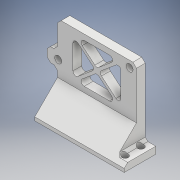
# Autodesk Inventor part: PingCover-y
Saved by Autodesk Inventor 2018.3 (Build 223284000, 284)
## iProperties
Created: 2018-08-25
Part Number: PingCover-y
Material: ABS プラスチック
Document SubType Name: Modeling
Designer: shun2
Density: 1.06 g/cm^3
Appearance: 滑らか - 白
Author: shun2
Autodesk Inventor part; units mm, degrees
sketch "スケッチ1" plane through (0, 0, 0) normal (0, 0, 1) x (1, 0, 0)
  line L0 (0, 0) -> (51, 0)
  line L1 (51, 0) -> (51, 18)
  line L2 (51, 18) -> (0, 18)
  line L3 (0, 18) -> (0, 0)
  circle A0 centre (47, 13.5) radius 1.8
  circle A1 centre (47, 4.5) radius 1.8
  dimension "d0" = 51
  dimension "d1" = 18
  dimension "d4" = 3.6
  dimension "d5" = 13.5
  dimension "d6" = 4
  dimension "d7" = 3.6
  dimension "d8" = 4
  dimension "d9" = 4.5
  constraints: 8 end point, 2 centre point, 2 parallel, 1 horizontal, 1 perpendicular
  measures "d0" distance of L2.end L1.end
  measures "d1" distance of L1.end L0.end
  measures "d4" diameter of A0
  measures "d5" distance from line of L0 A0.centre
  measures "d6" distance from line of L1 A0.centre
  measures "d7" diameter of A1
  measures "d8" distance from line of L1 A1.centre
  measures "d9" distance from line of L0 A1.centre
extrude "押し出し2" add sketch "スケッチ1" along normal blind 2
sketch "スケッチ2" plane through (0, 0, 2) normal (0, 0, 1) x (1, 0, 0)
  line L0 (0, 18) -> (0, 0) projected
  line L1 (0, 18) -> (44, 18)
  line L2 (44, 18) -> (44, 13)
  line L3 (44, 13) -> (0, 13)
  line L4 (0, 13) -> (0, 18)
  dimension "d12" = 44
  dimension "d13" = 5
  constraints: 8 end point, 2 parallel, 1 horizontal, 1 perpendicular
  measures "d12" distance of L2.end L3.end
  measures "d13" distance of L1.end L2.end
extrude "押し出し3" add sketch "スケッチ2" along normal blind 42
sketch "スケッチ3" plane through (0, 13, 2) normal (0, -1, 0) x (1, 0, 0)
  circle A0 centre (41.1, 3.5) radius 2
  line L0 (44, 0) -> (44, 42) projected
  line L1 (44, 0) -> (0, 0) projected
  circle A1 centre (0.4, 19.8) radius 2
  point P0 (0, -2)
  dimension "d16" = 4
  dimension "d17" = 2.9
  dimension "d18" = 3.5
  dimension "d27" = 4
  dimension "d28" = 40.7
  dimension "d29" = 16.3
  constraints: 2 centre point
  measures "d16" diameter of A0
  measures "d17" distance from line of L0 A0.centre
  measures "d18" distance from line of L1 A0.centre
  measures "d27" diameter of A1
  measures "d28" horizontal distance of A0.centre A1.centre
  measures "d29" vertical distance of A0.centre A1.centre
sketch "スケッチ4" plane through (0, 13, 2) normal (0, -1, 0) x (1, 0, 0)
  line L0 (8, 13.3) -> (-4, 13.3)
  line L1 (-4, 13.3) -> (-4, 24.3)
  line L2 (-4, 24.3) -> (8, 24.3)
  line L3 (8, 24.3) -> (8, 13.3)
  line L4 (44, 0) -> (0, 0) projected
  line L5 (44, 0) -> (44, 42) projected
  line L6 (0, 42) -> (44, 42) projected
  line L7 (0, 0) -> (0, 42) projected
  point P0 (0, -2)
  dimension "d19" = 13.3
  dimension "d20" = 36
  dimension "d25" = 11
  dimension "d26" = 12
  constraints: 8 end point, 2 parallel, 1 horizontal, 1 perpendicular
  measures "d19" distance between parallel lines of L0 L4
  measures "d20" distance between parallel lines of L5 L3
  measures "d25" distance between parallel lines of L0 L2
  measures "d26" distance between parallel lines of L1 L3
ref_plane "作業平面2" through (-4, 15.3, 26.3) normal (0, -1, 0) x (1, 0, 0)
sketch "スケッチ5" plane through (-4, 15.3, 26.3) normal (0, -1, 0) x (1, 0, 0)
  point P0 (4, -26.3)
ref_plane "作業平面1" through (-4, 15.3, 26.3) normal (0, -1, 0) x (1, 0, 0)
sketch "スケッチ6" plane through (-4, 15.3, 26.3) normal (0, -1, 0) x (1, 0, 0)
  line L0 (4, -24.3) -> (4, 17.7) projected
  circle A0 centre (4.4, -2.3) radius 2
  circle A1 centre (45.1, 14) radius 2
  line L1 (4, -24.3) -> (55, -24.3) projected
  line L2 (48, -24.3) -> (48, 17.7) projected
  line L3 (4, 17.7) -> (48, 17.7) projected
  point P0 (4, -26.3)
  dimension "d45" = 4
  dimension "d46" = 0.4
  dimension "d47" = 4
  dimension "d48" = 22
  dimension "d49" = 2.9
  dimension "d67" = 43.8427
  constraints: 2 centre point
  measures "d45" diameter of A0
  measures "d46" distance from line of L0 A0.centre
  measures "d47" diameter of A1
  measures "d48" distance from line of L1 A0.centre
  measures "d49" distance from line of L2 A1.centre
  measures "d67" distance of A0.centre A1.centre
sketch "スケッチ7" plane through (0, 13, 2) normal (0, -1, 0) x (1, 0, 0)
  point P0 (0, -2)
sketch "スケッチ8" plane through (0, 13, 2) normal (0, -1, 0) x (1, 0, 0)
  line L0 (44, 0) -> (44, 42) projected
  line L1 (44, 0) -> (45, 0)
  line L2 (45, 0) -> (45, 21.3)
  line L3 (45, 21.3) -> (44, 21.3)
  line L4 (44, 21.3) -> (44, 0)
  point P0 (0, -2)
  dimension "d35" = 1
  constraints: 8 end point, 2 parallel, 1 horizontal, 1 perpendicular
  measures "d35" distance of L3.end L2.end
extrude "押し出し6" add sketch "スケッチ8" against normal blind 5
ref_plane "作業平面3" through (45, 13, 3) normal (0, -1, 0) x (1, 0, 0)
sketch "スケッチ9" plane through (45, 13, 3) normal (0, -1, 0) x (1, 0, 0)
  line L0 (-51, 17.2309) -> (-43, 17.2309)
  line L1 (-43, 17.2309) -> (-43, 25.2309)
  line L2 (-43, 25.2309) -> (-51, 25.2309)
  line L3 (-51, 25.2309) -> (-51, 17.2309)
  line L4 (0, 41) -> (-10, 41)
  line L5 (-10, 41) -> (-10, 7.258)
  line L6 (-10, 7.258) -> (0, 7.258)
  line L7 (0, 7.258) -> (0, 41)
  line L8 (0, 16.7) -> (0, 41)
  line L9 (-45, -1) -> (6, -1) projected
  point P0 (-45, -3)
  point P1 (-45, 4.4596)
  point P2 (-2.5771, 20.3)
  dimension "d55" = 8
  dimension "d59" = 0
  dimension "d97" = 18.2309
  dimension "d98" = 8.258
  dimension "d99" = 33.742
  constraints: 18 end point, 2 parallel, 1 horizontal, 1 perpendicular
  measures "d55" distance between parallel lines of L0 L2
  measures "d59" distance between parallel lines of L8 L7
  measures "d97" distance between parallel lines of L0 L9
  measures "d98" distance between parallel lines of L6 L9
  measures "d99" distance between parallel lines of L4 L6
extrude "押し出し8" add sketch "スケッチ9" against normal blind 5
extrude "押し出し9" cut sketch "スケッチ6" along normal mid plane 10 contours A0 L0 | L0 A0 | A1
chamfer "面取り5" distance 13 angle 45 1 edges at (22.5, 13, 2)
sketch "スケッチ10" plane through (0, 0, 2) normal (0, 0, 1) x (1, 0, 0)
  line L0 (45, 18) -> (45, 0) projected
  line L1 (45, 0) -> (51, 0) projected
  line L2 (51, 0) -> (51, 18) projected
  line L3 (51, 18) -> (45, 18) projected
  circle A0 centre (47, 13.5) radius 1.8 projected
  circle A1 centre (47, 4.5) radius 1.8 projected
  circle A2 centre (47, 4.5) radius 1.8
  circle A3 centre (47, 13.5) radius 1.8
  line L4 (45, 0) -> (51, 0)
  line L5 (51, 0) -> (51, 18)
  line L6 (51, 18) -> (45, 18)
  line L7 (45, 18) -> (45, 0)
  point P0 (0, 0)
  constraints: 8 end point, 2 centre point, 2 coincident, 2 concentric, 2 parallel, 1 horizontal, 1 perpendicular
extrude "押し出し10" add sketch "スケッチ10" along normal blind 2
chamfer "面取り6" distance 2 angle 45 1 edges at (48, 0, 4)
chamfer "面取り7" distance 1.5 angle 45 1 edges at (45, 10.0001, 4)
chamfer "面取り8" distance 2 angle 45 4 edges at (45, 15.5, 44) (0, 15.5, 44) (-6, 15.5, 20.2309) (-6, 15.5, 28.2309)
sketch "スケッチ11" plane through (0, 13, 15) normal (0, -1, 0) x (1, 0, 0)
  line L0 (45, 0) -> (45, 27) projected
  line L1 (45, 13.5) -> (35.6998, 13.5)
  line L2 (19.8872, 15.8543) -> (11.6558, 22.7612)
  line L3 (21.4786, 14.5189) -> (32.2238, 14.5189) construction
  line L4 (19.8872, 13.1836) -> (11.6558, 6.2766)
  line L5 (21.4786, 14.5189) -> (32.2239, 14.5189) construction
  line L6 (8.7921, 7.612) -> (8.7921, 21.4259)
  arc A0 (11.6558, 22.7612) -> (8.7921, 21.4259) centre (10.5353, 21.4258) ccw
  arc A1 (19.8872, 13.1836) -> (19.8872, 15.8543) centre (18.7667, 14.5189) ccw
  arc A2 (8.7921, 7.612) -> (11.6558, 6.2766) centre (10.5353, 7.612) ccw
  line L7 (25.0769, 15.8544) -> (33.3082, 22.7613)
  line L8 (25.0769, 13.1835) -> (33.3082, 6.2766)
  line L9 (36.1721, 7.612) -> (36.1721, 21.4258)
  arc A3 (36.1721, 21.4258) -> (33.3082, 22.7613) centre (34.4288, 21.4258) ccw
  arc A4 (25.0769, 15.8544) -> (25.0769, 13.1835) centre (26.1975, 14.5189) ccw
  arc A5 (33.3082, 6.2766) -> (36.1721, 7.612) centre (34.4288, 7.612) ccw
  line L10 (23.55, 16.7078) -> (30.7794, 22.774)
  line L11 (23.8988, 16.5352) -> (33.3361, 16.5352) construction
  line L12 (21.3092, 16.7078) -> (14.0798, 22.774)
  line L13 (23.8988, 16.5352) -> (33.3361, 16.5352) construction
  line L14 (15.2002, 25.8522) -> (29.659, 25.8522)
  arc A6 (21.3092, 16.7078) -> (23.55, 16.7078) centre (22.4296, 18.043) ccw
  arc A7 (15.2002, 25.8522) -> (14.0798, 22.774) centre (15.2002, 24.1092) ccw
  arc A8 (30.7794, 22.774) -> (29.659, 25.8522) centre (29.659, 24.1092) ccw
  line L15 (23.5502, 12.3302) -> (30.7795, 6.2641)
  line L16 (21.309, 12.3302) -> (14.0797, 6.2641)
  line L17 (15.2003, 3.1853) -> (29.6589, 3.1853)
  arc A9 (23.5502, 12.3302) -> (21.309, 12.3302) centre (22.4296, 10.9947) ccw
  arc A10 (14.0797, 6.2641) -> (15.2003, 3.1853) centre (15.2003, 4.9286) ccw
  arc A11 (29.6589, 3.1853) -> (30.7795, 6.2641) centre (29.6589, 4.9286) ccw
  point P0 (0, -15)
  point P1 (8.7921, 25.1641)
  point P2 (8.792, 3.8737)
  point P3 (23.4854, 14.5189)
  point P4 (36.1721, 25.1643)
  point P5 (36.1721, 3.8735)
  point P6 (35.918, 26.6205)
  point P7 (11.8795, 26.6205)
  point P8 (21.9006, 14.5189)
  dimension "d82" = 16.561
  dimension "d83" = 140
  dimension "d84" = 16.5611
  dimension "d85" = 140
  dimension "d86" = 1.7432
  dimension "d87" = 15.69
  dimension "d88" = 40
  dimension "d89" = 15.69
  dimension "d90" = 140
  dimension "d91" = 1.743
  constraints: 34 end point, 24 point on circle, 12 centre point, 12 point on line, 12 tangent, 5 horizontal, 4 equal length, 4 equal radius, 1 midpoint
  measures "d82" distance of L3.start point (8.792, 25.164)
  measures "d83" angle of L3 L2
  measures "d84" distance of L3.start point (8.792, 3.874)
  measures "d85" angle of L4 L5
  measures "d86" radius of A0
  measures "d87" distance of L11.start point (35.918, 26.621)
  measures "d88" angle of L11 L10
  measures "d89" distance of L11.start point (11.88, 26.621)
  measures "d90" angle of L13 L12
  measures "d91" radius of A6
extrude "押し出し11" cut sketch "スケッチ11" against normal blind 5
chamfer "面取り9" distance 2 angle 45 2 edges at (0, 15.5, 28.2309) (0, 15.5, 20.2309)
